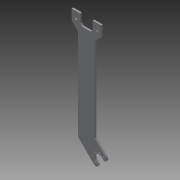
# Autodesk Inventor part: Arm_Link
Saved by Autodesk Inventor 2013 (Build 170138000, 138)
## iProperties
Created: 2014-05-07
Part Number: Arm_Link
Material: 一般
Document SubType Name: Modeling
Designer: andou
Density: 1 g/cm^3
Author: andou
Autodesk Inventor part; units mm, degrees
ref_plane "YZ Plane" through (0, 0, 0) normal (1, 0, 0) x (0, 1, 0)
ref_plane "XZ Plane" through (0, 0, 0) normal (0, 1, 0) x (-1, 0, 0)
ref_plane "XY Plane" through (0, 0, 0) normal (0, 0, 1) x (1, 0, 0)
sketch "スケッチ1" plane through (0, 0, 0) normal (0, 1, 0) x (-1, 0, 0)
  line L0 (-17.5, 70) -> (-7.5, 70)
  line L1 (-7.5, 70) -> (-7.5, 60)
  line L2 (-7.5, 60) -> (-5, 57.5)
  line L3 (-5, 57.5) -> (5, 57.5)
  line L4 (5, 57.5) -> (7.5, 60)
  line L5 (7.5, 60) -> (7.5, 70)
  line L6 (7.5, 70) -> (17.5, 70)
  circle A0 centre (-12.5, 62.5) radius 1.5
  circle A1 centre (12.5, 62.5) radius 1.5
  line L7 (-17.5, 70) -> (-17.5, 57.5)
  line L8 (-17.5, 57.5) -> (-10, 50)
  line L9 (17.5, 70) -> (17.5, 57.5)
  line L10 (17.5, 57.5) -> (10, 50)
  line L11 (-10, 50) -> (-10, -50)
  line L12 (-10, -50) -> (-25.3553, -65.3553)
  line L13 (-11.2132, -79.4975) -> (10, -58.2843)
  line L14 (10, -58.2843) -> (10, 50)
  line L15 (0, 0) -> (47.4517, 0)
  line L16 (-21.8198, -68.8909) -> (-18.2843, -65.3553)
  line L17 (-11.2132, -72.4264) -> (-14.7487, -75.9619)
  arc A2 (-11.2132, -72.4264) -> (-18.2843, -65.3553) centre (-14.7487, -68.8909) ccw
  line L18 (-25.3553, -65.3553) -> (-21.8198, -68.8909)
  line L19 (-14.7487, -75.9619) -> (-11.2132, -79.4975)
  dimension "d2" = 10
  dimension "d3" = 135
  dimension "d4" = 45
  dimension "d6" = 15
  dimension "d7" = 2.5
  dimension "d8" = 10
  dimension "d9" = 10
  dimension "d10" = 10
  dimension "d11" = 10
  dimension "d12" = 90
  dimension "d15" = 25
  dimension "d16" = 5
  dimension "d17" = 20
  dimension "d18" = 7.5
  dimension "d19" = 7.5
  dimension "d20" = 5
  dimension "d21" = 100
  dimension "d22" = 20
  dimension "d23" = 135
  dimension "d24" = 10
  dimension "d27" = 20
  dimension "d28" = 50
  dimension "d29" = 90
  dimension "d31" = 3
  dimension "d33" = 10
  dimension "d35" = 10
  dimension "d37" = 5
  dimension "d38" = 5
  dimension "d39" = 5
  dimension "d40" = 30
  constraints: 40 end point, 7 perpendicular, 6 parallel, 3 centre point, 2 equal length, 2 point on circle, 1 collinear, 1 equal radius, 1 horizontal
  measures "d2" distance of L2.end L3.end
  measures "d3" angle of L3 L2
  measures "d4" angle of L4 L3
  measures "d6" distance between parallel lines of L5 L1
  measures "d7" distance from line of L5 L3.end
  measures "d8" distance of L4.end L5.end
  measures "d9" distance of L0.end L1.end
  measures "d10" distance of L0.start L0.end
  measures "d11" distance of L5.end L6.end
  measures "d12" angle of L0 L1
  measures "d15" distance of A1.centre A0.centre
  measures "d16" distance from line of L1 A0.centre
  measures "d17" distance of L10.end L8.end
  measures "d18" distance from line of L0 A0.centre
  measures "d19" distance from line of L6 A1.centre
  measures "d20" distance from line of L9 A1.centre
  measures "d21" distance of L8.end L11.end
  measures "d22" distance between parallel lines of L13 L12
  measures "d23" angle of L11 L12
  measures "d24" distance from line of L14 L15.start
  measures "d27" distance from line of L6 L10.end
  measures "d28" vertical distance of L15.start L10.end
  measures "d29" angle of L14 L15
  measures "d31" diameter of A1
  measures "d33" distance between parallel lines of L17 L16
  measures "d35" distance from line of L13 A2.centre
  measures "d37" radius of A2
  measures "d38" distance from line of L19 A2.centre
  measures "d39" distance from line of A2.centre L18
  measures "d40" distance of L13.start L13.end
extrude "押し出し2" add sketch "スケッチ1" along normal blind 2
sketch "スケッチ2" plane through (0, 2, 0) normal (0, 1, 0) x (1, 0, 0)
  line L0 (25.3553, 65.3553) -> (21.8198, 68.8909) projected
  arc A0 (11.2132, 72.4264) -> (18.2843, 65.3553) centre (14.7487, 68.8909) ccw projected
  circle A1 centre (19.6985, 63.9411) radius 1
  point P0 (0, 0)
  dimension "d48" = 5
  dimension "d49" = 7
  dimension "d50" = 2
  constraints: 1 centre point
  measures "d48" distance from line of L0 A1.centre
  measures "d49" distance of A0.centre A1.centre
  measures "d50" diameter of A1
hole "穴1" at (19.6985, 2, -63.9411) direction (0, -1, 0) diameter 2 end through all
pattern_circular "円形状パターン1" count 5 over 180 about axis through (14.7487, 0, -68.8909) along (0, -1, 0) of "穴1"
sketch "スケッチ3" plane through (0, 2, 0) normal (0, 1, 0) x (1, 0, 0)
  circle A0 centre (9.799, 73.8406) radius 1 projected
  circle A1 centre (7.7487, 68.8909) radius 1 projected
  circle A2 centre (9.799, 63.9411) radius 1 projected
  circle A3 centre (14.7487, 61.8909) radius 1 projected
  circle A4 centre (19.6985, 63.9411) radius 1 projected
  circle A5 centre (-12.5, -62.5) radius 1.5 projected
  circle A6 centre (12.5, -62.5) radius 1.5 projected
  line L0 (7.5, -70) -> (17.5, -70) projected
  line L1 (17.5, -70) -> (17.5, -57.5) projected
  line L2 (17.5, -57.5) -> (10, -50) projected
  line L3 (10, -50) -> (10, 50) projected
  line L4 (10, 50) -> (25.3553, 65.3553) projected
  line L5 (25.3553, 65.3553) -> (21.8198, 68.8909) projected
  line L6 (21.8198, 68.8909) -> (18.2843, 65.3553) projected
  arc A7 (11.2132, 72.4264) -> (18.2843, 65.3553) centre (14.7487, 68.8909) ccw projected
  line L7 (11.2132, 72.4264) -> (14.7487, 75.9619) projected
  line L8 (14.7487, 75.9619) -> (11.2132, 79.4975) projected
  line L9 (11.2132, 79.4975) -> (-10, 58.2843) projected
  line L10 (-10, 58.2843) -> (-10, -50) projected
  line L11 (-10, -50) -> (-17.5, -57.5) projected
  line L12 (-17.5, -57.5) -> (-17.5, -70) projected
  line L13 (-17.5, -70) -> (-7.5, -70) projected
  line L14 (-7.5, -70) -> (-7.5, -60) projected
  line L15 (-7.5, -60) -> (-5, -57.5) projected
  line L16 (-5, -57.5) -> (5, -57.5) projected
  line L17 (5, -57.5) -> (7.5, -60) projected
  line L18 (7.5, -60) -> (7.5, -70) projected
  arc A8 (12.1605, 78.5501) -> (7.6777, 75.9619) centre (14.7487, 68.8909) ccw
  arc A9 (21.8198, 61.8198) -> (24.408, 66.3027) centre (14.7487, 68.8909) ccw
  point P0 (0, 0)
  constraints: 4 point on circle, 4 point on line, 2 centre point, 1 coincident, 1 concentric, 1 tangent
extrude "押し出し3" cut sketch "スケッチ3" against normal blind 2 contours L18 L17 L16 L15 L14 L13 L12 L11 L10 L9 A8 L8 L7 A7 L6 L5 A9 L4 L3 L2 L1 L0 keep common part
fillet "フィレット1" radius 2 4 edges at (14.7487, 1, -75.9619) (21.8198, 1, -68.8909) (24.408, 1, -66.3027) (12.1605, 1, -78.5501)
fillet "フィレット2" radius 2 4 edges at (-5, 1, 57.5) (-7.5, 1, 60) (5, 1, 57.5) (7.5, 1, 60)
